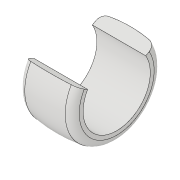
# Autodesk Inventor part: 11_027_SHOE_GRIP_RUBBER_R1
Saved by Autodesk Inventor 2021.2 (Build 252289000, 289)
## iProperties
Created: 2020-02-11
Part Number: 11_027_SHOE_GRIP_RUBBER_R1
Material: ゴム、シリコーン
Document SubType Name: Modeling
Designer: y6tada
Density: 1.25 g/cm^3
Appearance: 滑らか - 白
Mass: 2.34526 g
Surface Area: 14.823 cm^2
Volume: 1.87621 cm^3
Author: y6tada
Autodesk Inventor part; units mm, degrees
ref_plane "YZ Plane" through (0, 0, 0) normal (1, 0, 0) x (0, 1, 0)
ref_plane "XZ Plane" through (0, 0, 0) normal (0, 1, 0) x (-1, 0, 0)
ref_plane "XY Plane" through (0, 0, 0) normal (0, 0, 1) x (1, 0, 0)
sketch "スケッチ1" plane through (0, 0, 0) normal (0, 0, 1) x (1, 0, 0)
  line L0 (0, 0) -> (23.2776, 0) construction
  line L1 (-7, -8.8) -> (7, -8.8)
  line L2 (7, -8.8) -> (7, -11.5)
  line L3 (7, -11.5) -> (-7, -11.5) construction
  line L4 (-7, -11.5) -> (-7, -8.8)
  line L5 (0, 0) -> (0, -16.4759) construction
  arc A0 (-7, -11.5) -> (7, -11.5) centre (0, 23.15) ccw
  line L6 (0, -12.2) -> (12.7013, -12.2) construction
  line L7 (0, 0) -> (-18.8146, 0) construction
  dimension "d0" = 14
  dimension "d1" = 8.8
  dimension "d2" = 12.2
  dimension "d4" = 11.5
  constraints: 16 end point, 4 horizontal, 3 point on circle, 2 parallel, 1 centre point, 1 perpendicular, 1 vertical, 1 other
  measures "d0" distance between parallel lines of L4 L2
  measures "d1" distance between parallel lines of L0 L1
  measures "d2" distance between parallel lines of L0 L6
  measures "d4" distance between parallel lines of L0 L3
revolve "回転1" add sketch "スケッチ1" angle 240 mid plane about axis through (0, 0, 0) along (-1, 0, 0)
fillet "フィレット1" radius 2 2 edges at (7, -11.5, 0) (-7, -11.5, 0)
